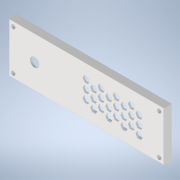
# Autodesk Inventor part: A-04
Saved by Autodesk Inventor 2022.2 (Build 262287000, 287)
## iProperties
Created: 2021-11-25
Part Number: A-04
Material: Generic
Document SubType Name: Modeling
Designer: kfcs7
Density: 1 g/cm^3
Appearance: Default
Author: kfcs7
Autodesk Inventor part; units mm, degrees
ref_plane "YZ Plane" through (0, 0, 0) normal (1, 0, 0) x (0, 1, 0)
ref_plane "XZ Plane" through (0, 0, 0) normal (0, 1, 0) x (-1, 0, 0)
ref_plane "XY Plane" through (0, 0, 0) normal (0, 0, 1) x (1, 0, 0)
sketch "Sketch1" plane through (0, 0, 0) normal (0, 0, 1) x (1, 0, 0)
  circle A0 centre (4, 4) radius 2.25 construction
  line L0 (119, 20) -> (119, 10.0711) construction
  line L1 (119, 10.0711) -> (113.9289, 5) construction
  line L2 (113.9289, 5) -> (10.0711, 5) construction
  line L3 (10.0711, 5) -> (5, 10.0711) construction
  line L4 (5, 10.0711) -> (5, 20) construction
  line L5 (0, 20) -> (5, 20) construction
  line L6 (0, 0) -> (0, 20) construction
  line L7 (124, 0) -> (0, 0) construction
  line L8 (124, 0) -> (124, 20) construction
  line L9 (119, 20) -> (124, 20) construction
  circle A1 centre (120, 4) radius 2.25 construction
  circle A2 centre (120, 36) radius 2.25 construction
  line L10 (119, 29.9289) -> (119, 20) construction
  line L11 (124, 20) -> (119, 20) construction
  line L12 (124, 40) -> (124, 20) construction
  line L13 (0, 40) -> (124, 40) construction
  line L14 (0, 20) -> (0, 40) construction
  line L15 (5, 20) -> (0, 20) construction
  line L16 (5, 20) -> (5, 29.9289) construction
  line L17 (5, 29.9289) -> (10.0711, 35) construction
  line L18 (10.0711, 35) -> (113.9289, 35) construction
  line L19 (113.9289, 35) -> (119, 29.9289) construction
  circle A3 centre (4, 36) radius 2.25 construction
  line L20 (124, 0) -> (0, 0)
  line L21 (0, 0) -> (0, 40)
  line L22 (0, 40) -> (124, 40)
  line L23 (124, 40) -> (124, 0)
  constraints: 8 end point, 2 parallel, 1 horizontal, 1 perpendicular
extrude "Extrusion1" add sketch "Sketch1" along normal blind 6 draft -5
sketch "Sketch4" plane through (0, 0, 0) normal (0, 0, -1) x (-1, 0, 0)
  line L0 (-124, 40) -> (0, 40) construction
  line L1 (-124, 0) -> (-124, 40) construction
  line L2 (0, 0) -> (-124, 0) construction
  line L3 (0, 40) -> (0, 0) construction
  circle A0 centre (-120, 4) radius 2.25 construction
  line L4 (-119, 10.0711) -> (-119, 20) projected
  line L5 (-124, 20) -> (-119, 20) construction
  line L6 (-124, 0) -> (-124, 20) construction
  line L7 (0, 0) -> (-124, 0) construction
  line L8 (0, 20) -> (0, 0) construction
  line L9 (-5, 20) -> (0, 20) construction
  line L10 (-5, 20) -> (-5, 10.0711) projected
  line L11 (-5, 10.0711) -> (-10.0711, 5) projected
  line L12 (-10.0711, 5) -> (-113.9289, 5) projected
  line L13 (-113.9289, 5) -> (-119, 10.0711) projected
  circle A1 centre (-4, 4) radius 2.25 construction
  circle A2 centre (-4, 36) radius 2.25 construction
  line L14 (-119, 20) -> (-119, 29.9289) projected
  line L15 (-119, 29.9289) -> (-113.9289, 35) projected
  line L16 (-113.9289, 35) -> (-10.0711, 35) projected
  line L17 (-10.0711, 35) -> (-5, 29.9289) projected
  line L18 (-5, 29.9289) -> (-5, 20) projected
  line L19 (0, 20) -> (-5, 20) construction
  line L20 (0, 40) -> (0, 20) construction
  line L21 (-124, 40) -> (0, 40) construction
  line L22 (-124, 40) -> (-124, 20) construction
  line L23 (-119, 20) -> (-124, 20) construction
  circle A3 centre (-120, 36) radius 2.25 construction
extrude "Extrusion4" cut sketch "Sketch4" against normal blind 4.5 draft -25
sketch "Sketch5" plane through (0, 0, 6) normal (0, 0, 1) x (1, 0, 0)
  circle A0 centre (120, 4) radius 1.7718 projected
  circle A1 centre (120, 36) radius 1.7718 projected
  circle A2 centre (4, 36) radius 1.7718 projected
  circle A3 centre (4, 4) radius 1.7718 projected
  point P0 (0, 0)
extrude "Extrusion5" cut sketch "Sketch5" against normal through all
sketch "Sketch6" plane through (0, 0, 6) normal (0, 0, 1) x (1, 0, 0)
  circle A0 centre (120, 4) radius 1.7718 projected
  circle A1 centre (4, 36) radius 1.7718 projected
  circle A2 centre (120, 36) radius 1.7718 projected
  circle A3 centre (4, 4) radius 1.7718 projected
  line L0 (123.4751, 39.4751) -> (123.4751, 0.5249) projected
  line L1 (0.5249, 39.4751) -> (123.4751, 39.4751) projected
  line L2 (0.5249, 0.5249) -> (0.5249, 39.4751) projected
  line L3 (123.4751, 0.5249) -> (0.5249, 0.5249) projected
  line L4 (60.5566, 24.25) -> (63.4434, 24.25)
  line L5 (63.4434, 24.25) -> (64.8868, 21.75)
  line L6 (64.8868, 21.75) -> (63.4434, 19.25)
  line L7 (63.4434, 19.25) -> (60.5566, 19.25)
  line L8 (60.5566, 19.25) -> (59.1133, 21.75)
  line L9 (59.1133, 21.75) -> (60.5566, 24.25)
  line L10 (66.6188, 20.75) -> (69.5056, 20.75)
  line L11 (69.5056, 20.75) -> (70.9489, 18.25)
  line L12 (70.9489, 18.25) -> (69.5056, 15.75)
  line L13 (69.5056, 15.75) -> (66.6188, 15.75)
  line L14 (66.6188, 15.75) -> (65.1754, 18.25)
  line L15 (65.1754, 18.25) -> (66.6188, 20.75)
  line L16 (123.4751, 0.5249) -> (0.5249, 0.5249) projected
  line L17 (68.0622, 18.25) -> (62, 21.75) construction
  line L18 (123.4751, 39.4751) -> (123.4751, 0.5249) projected
  point P0 (0, 0)
  point P1 (65.0311, 20)
  dimension "d35" = 5
  dimension "d36" = 5
  dimension "d37" = 2
  dimension "d39" = 38.9501
  dimension "d40" = 122.9501
  dimension "d41" = 61.4751
  dimension "d46" = 19.4751
  constraints: 26 end point, 2 parallel, 1 midpoint, 1 perpendicular, 26 other
  measures "d35" distance between parallel lines of L7 L4
  measures "d36" distance between parallel lines of L13 L10
  measures "d37" distance between parallel lines of L6 L15
  measures "d39" distance of L2.start L1.start
  measures "d40" distance of L0.end L2.start
  measures "d41" distance from line of L2 L17.end
  measures "d46" distance from line of L3 point (65.031, 20)
extrude "Extrusion6" cut sketch "Sketch6" against normal through all contours L4 L5 L6 L7 L8 L9 | L10 L11 L12 L13 L14 L15
pattern_linear "Rectangular Pattern1" count 4 spacing 12 along (1, 0, 0) count 3 spacing 7 along (0, -1, 0) of "Extrusion6" second direction both ways yes
sketch "Sketch7" plane through (0, 0, 6) normal (0, 0, 1) x (1, 0, 0)
  line L0 (96.5566, 17.25) -> (99.4434, 17.25) projected
  line L1 (99.4434, 17.25) -> (100.8868, 14.75) projected
  line L2 (100.8868, 14.75) -> (99.4434, 12.25) projected
  line L3 (99.4434, 12.25) -> (96.5566, 12.25) projected
  line L4 (96.5566, 12.25) -> (95.1133, 14.75) projected
  line L5 (95.1133, 14.75) -> (96.5566, 17.25) projected
  line L6 (105.5056, 13.75) -> (106.9489, 11.25) projected
  line L7 (106.9489, 11.25) -> (105.5056, 8.75) projected
  line L8 (105.5056, 8.75) -> (102.6188, 8.75) projected
  line L9 (102.6188, 8.75) -> (101.1754, 11.25) projected
  line L10 (101.1754, 11.25) -> (102.6188, 13.75) projected
  line L11 (102.6188, 13.75) -> (105.5056, 13.75) projected
  line L12 (84.5566, 17.25) -> (87.4434, 17.25) projected
  line L13 (87.4434, 17.25) -> (88.8868, 14.75) projected
  line L14 (88.8868, 14.75) -> (87.4434, 12.25) projected
  line L15 (87.4434, 12.25) -> (84.5566, 12.25) projected
  line L16 (84.5566, 12.25) -> (83.1133, 14.75) projected
  line L17 (83.1133, 14.75) -> (84.5566, 17.25) projected
  line L18 (93.5056, 13.75) -> (94.9489, 11.25) projected
  line L19 (94.9489, 11.25) -> (93.5056, 8.75) projected
  line L20 (93.5056, 8.75) -> (90.6188, 8.75) projected
  line L21 (90.6188, 8.75) -> (89.1754, 11.25) projected
  line L22 (89.1754, 11.25) -> (90.6188, 13.75) projected
  line L23 (90.6188, 13.75) -> (93.5056, 13.75) projected
  line L24 (72.5566, 17.25) -> (75.4434, 17.25) projected
  line L25 (75.4434, 17.25) -> (76.8868, 14.75) projected
  line L26 (76.8868, 14.75) -> (75.4434, 12.25) projected
  line L27 (75.4434, 12.25) -> (72.5566, 12.25) projected
  line L28 (72.5566, 12.25) -> (71.1133, 14.75) projected
  line L29 (71.1133, 14.75) -> (72.5566, 17.25) projected
  line L30 (81.5056, 13.75) -> (82.9489, 11.25) projected
  line L31 (82.9489, 11.25) -> (81.5056, 8.75) projected
  line L32 (81.5056, 8.75) -> (78.6188, 8.75) projected
  line L33 (78.6188, 8.75) -> (77.1754, 11.25) projected
  line L34 (77.1754, 11.25) -> (78.6188, 13.75) projected
  line L35 (78.6188, 13.75) -> (81.5056, 13.75) projected
  line L36 (60.5566, 17.25) -> (63.4434, 17.25) projected
  line L37 (63.4434, 17.25) -> (64.8868, 14.75) projected
  line L38 (64.8868, 14.75) -> (63.4434, 12.25) projected
  line L39 (63.4434, 12.25) -> (60.5566, 12.25) projected
  line L40 (60.5566, 12.25) -> (59.1133, 14.75) projected
  line L41 (59.1133, 14.75) -> (60.5566, 17.25) projected
  line L42 (69.5056, 13.75) -> (70.9489, 11.25) projected
  line L43 (70.9489, 11.25) -> (69.5056, 8.75) projected
  line L44 (69.5056, 8.75) -> (66.6188, 8.75) projected
  line L45 (66.6188, 8.75) -> (65.1754, 11.25) projected
  line L46 (65.1754, 11.25) -> (66.6188, 13.75) projected
  line L47 (66.6188, 13.75) -> (69.5056, 13.75) projected
  line L48 (96.5566, 24.25) -> (99.4434, 24.25) projected
  line L49 (99.4434, 24.25) -> (100.8868, 21.75) projected
  line L50 (100.8868, 21.75) -> (99.4434, 19.25) projected
  line L51 (99.4434, 19.25) -> (96.5566, 19.25) projected
  line L52 (96.5566, 19.25) -> (95.1133, 21.75) projected
  line L53 (95.1133, 21.75) -> (96.5566, 24.25) projected
  line L54 (105.5056, 20.75) -> (106.9489, 18.25) projected
  line L55 (106.9489, 18.25) -> (105.5056, 15.75) projected
  line L56 (105.5056, 15.75) -> (102.6188, 15.75) projected
  line L57 (102.6188, 15.75) -> (101.1754, 18.25) projected
  line L58 (101.1754, 18.25) -> (102.6188, 20.75) projected
  line L59 (102.6188, 20.75) -> (105.5056, 20.75) projected
  line L60 (84.5566, 24.25) -> (87.4434, 24.25) projected
  line L61 (87.4434, 24.25) -> (88.8868, 21.75) projected
  line L62 (88.8868, 21.75) -> (87.4434, 19.25) projected
  line L63 (87.4434, 19.25) -> (84.5566, 19.25) projected
  line L64 (84.5566, 19.25) -> (83.1133, 21.75) projected
  line L65 (83.1133, 21.75) -> (84.5566, 24.25) projected
  line L66 (93.5056, 20.75) -> (94.9489, 18.25) projected
  line L67 (94.9489, 18.25) -> (93.5056, 15.75) projected
  line L68 (93.5056, 15.75) -> (90.6188, 15.75) projected
  line L69 (90.6188, 15.75) -> (89.1754, 18.25) projected
  line L70 (89.1754, 18.25) -> (90.6188, 20.75) projected
  line L71 (90.6188, 20.75) -> (93.5056, 20.75) projected
  line L72 (72.5566, 24.25) -> (75.4434, 24.25) projected
  line L73 (75.4434, 24.25) -> (76.8868, 21.75) projected
  line L74 (76.8868, 21.75) -> (75.4434, 19.25) projected
  line L75 (75.4434, 19.25) -> (72.5566, 19.25) projected
  line L76 (72.5566, 19.25) -> (71.1133, 21.75) projected
  line L77 (71.1133, 21.75) -> (72.5566, 24.25) projected
  line L78 (81.5056, 20.75) -> (82.9489, 18.25) projected
  line L79 (82.9489, 18.25) -> (81.5056, 15.75) projected
  line L80 (81.5056, 15.75) -> (78.6188, 15.75) projected
  line L81 (78.6188, 15.75) -> (77.1754, 18.25) projected
  line L82 (77.1754, 18.25) -> (78.6188, 20.75) projected
  line L83 (78.6188, 20.75) -> (81.5056, 20.75) projected
  line L84 (96.5566, 31.25) -> (99.4434, 31.25) projected
  line L85 (99.4434, 31.25) -> (100.8868, 28.75) projected
  line L86 (100.8868, 28.75) -> (99.4434, 26.25) projected
  line L87 (99.4434, 26.25) -> (96.5566, 26.25) projected
  line L88 (96.5566, 26.25) -> (95.1133, 28.75) projected
  line L89 (95.1133, 28.75) -> (96.5566, 31.25) projected
  line L90 (105.5056, 27.75) -> (106.9489, 25.25) projected
  line L91 (106.9489, 25.25) -> (105.5056, 22.75) projected
  line L92 (105.5056, 22.75) -> (102.6188, 22.75) projected
  line L93 (102.6188, 22.75) -> (101.1754, 25.25) projected
  line L94 (101.1754, 25.25) -> (102.6188, 27.75) projected
  line L95 (102.6188, 27.75) -> (105.5056, 27.75) projected
  line L96 (84.5566, 31.25) -> (87.4434, 31.25) projected
  line L97 (87.4434, 31.25) -> (88.8868, 28.75) projected
  line L98 (88.8868, 28.75) -> (87.4434, 26.25) projected
  line L99 (87.4434, 26.25) -> (84.5566, 26.25) projected
  line L100 (84.5566, 26.25) -> (83.1133, 28.75) projected
  line L101 (83.1133, 28.75) -> (84.5566, 31.25) projected
  line L102 (93.5056, 27.75) -> (94.9489, 25.25) projected
  line L103 (94.9489, 25.25) -> (93.5056, 22.75) projected
  line L104 (93.5056, 22.75) -> (90.6188, 22.75) projected
  line L105 (90.6188, 22.75) -> (89.1754, 25.25) projected
  line L106 (89.1754, 25.25) -> (90.6188, 27.75) projected
  line L107 (90.6188, 27.75) -> (93.5056, 27.75) projected
  line L108 (72.5566, 31.25) -> (75.4434, 31.25) projected
  line L109 (75.4434, 31.25) -> (76.8868, 28.75) projected
  line L110 (76.8868, 28.75) -> (75.4434, 26.25) projected
  line L111 (75.4434, 26.25) -> (72.5566, 26.25) projected
  line L112 (72.5566, 26.25) -> (71.1133, 28.75) projected
  line L113 (71.1133, 28.75) -> (72.5566, 31.25) projected
  line L114 (81.5056, 27.75) -> (82.9489, 25.25) projected
  line L115 (82.9489, 25.25) -> (81.5056, 22.75) projected
  line L116 (81.5056, 22.75) -> (78.6188, 22.75) projected
  line L117 (78.6188, 22.75) -> (77.1754, 25.25) projected
  line L118 (77.1754, 25.25) -> (78.6188, 27.75) projected
  line L119 (78.6188, 27.75) -> (81.5056, 27.75) projected
  line L120 (60.5566, 31.25) -> (63.4434, 31.25) projected
  line L121 (63.4434, 31.25) -> (64.8868, 28.75) projected
  line L122 (64.8868, 28.75) -> (63.4434, 26.25) projected
  line L123 (63.4434, 26.25) -> (60.5566, 26.25) projected
  line L124 (60.5566, 26.25) -> (59.1133, 28.75) projected
  line L125 (59.1133, 28.75) -> (60.5566, 31.25) projected
  line L126 (69.5056, 27.75) -> (70.9489, 25.25) projected
  line L127 (70.9489, 25.25) -> (69.5056, 22.75) projected
  line L128 (69.5056, 22.75) -> (66.6188, 22.75) projected
  line L129 (66.6188, 22.75) -> (65.1754, 25.25) projected
  line L130 (65.1754, 25.25) -> (66.6188, 27.75) projected
  line L131 (66.6188, 27.75) -> (69.5056, 27.75) projected
  line L132 (63.4434, 19.25) -> (60.5566, 19.25) projected
  line L133 (60.5566, 19.25) -> (59.1133, 21.75) projected
  line L134 (59.1133, 21.75) -> (60.5566, 24.25) projected
  line L135 (60.5566, 24.25) -> (63.4434, 24.25) projected
  line L136 (63.4434, 24.25) -> (64.8868, 21.75) projected
  line L137 (64.8868, 21.75) -> (63.4434, 19.25) projected
  line L138 (69.5056, 15.75) -> (66.6188, 15.75) projected
  line L139 (66.6188, 15.75) -> (65.1754, 18.25) projected
  line L140 (65.1754, 18.25) -> (66.6188, 20.75) projected
  line L141 (66.6188, 20.75) -> (69.5056, 20.75) projected
  line L142 (69.5056, 20.75) -> (70.9489, 18.25) projected
  line L143 (70.9489, 18.25) -> (69.5056, 15.75) projected
  circle A0 centre (120, 4) radius 1.7718 projected
  circle A1 centre (4, 36) radius 1.7718 projected
  circle A2 centre (120, 36) radius 1.7718 projected
  circle A3 centre (4, 4) radius 1.7718 projected
  line L144 (123.4751, 39.4751) -> (123.4751, 0.5249) projected
  line L145 (0.5249, 39.4751) -> (123.4751, 39.4751) projected
  line L146 (0.5249, 0.5249) -> (0.5249, 39.4751) projected
  line L147 (123.4751, 0.5249) -> (0.5249, 0.5249) projected
  circle A4 centre (21.0166, 20) radius 3.75
  point P0 (0, 0)
  dimension "d47" = 7.5
  dimension "d49" = 38.9501
  dimension "d50" = 19.4751
  dimension "d51" = 122.9501
  dimension "d52" = 20.4917
  constraints: 1 centre point
  measures "d47" diameter of A4
  measures "d49" distance of L146.start L145.start
  measures "d50" distance from line of L147 A4.centre
  measures "d51" distance of L144.end L146.start
  measures "d52" distance from line of L146 A4.centre
extrude "Extrusion7" cut sketch "Sketch7" against normal through all contours A4
fillet "Fillet1" radius 0.5 4 edges at (62, 0.5249, 6) (123.4751, 20, 6) (62, 39.4751, 6) (0.5249, 20, 6)
equation "\"d36\" = d35"
equation "\"d41\" = 0.5 * d40"
equation "\"d46\" = 0.5 * d39"
equation "\"d50\" = 0.5 * d49"
equation "\"d52\" = 0.166667 * d51"
body "Solid1"
